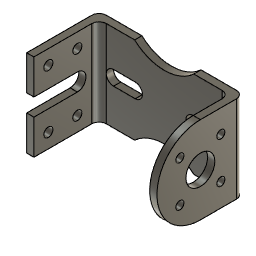
Tarea09_Ej2_jaalobuela (Autodesk Fusion 360 design; units mm, degrees)
Autodesk Fusion 360 part; units mm, degrees
sketch "Sketch1" plane through (0, 0, 0) normal (1, 0, 0) x (0, 1, 0)
  line L0 (-24.0301, 61.9141) -> (25.9699, 61.9141)
  line L1 (25.9699, 61.9141) -> (25.9699, 1.9141)
  line L2 (25.9699, 1.9141) -> (-24.0301, 1.9141)
  line L3 (-24.0301, 1.9141) -> (-29, 1.9141) construction
  line L4 (5.9699, 37.9141) -> (-24.0301, 37.9141)
  line L5 (5.9699, 25.9141) -> (-24.0301, 25.9141)
  arc A0 (5.9699, 25.9141) -> (5.9699, 37.9141) centre (5.9699, 31.9141) ccw
  line L6 (-24.0301, 1.9141) -> (-24.0301, 25.9141)
  line L7 (-24.0301, 37.9141) -> (-24.0301, 61.9141)
  line L8 (-24.0301, 61.9141) -> (-28, 61.9141) construction
  circle A1 centre (5.9699, 51.9141) radius 3.15
  circle A2 centre (-14.0301, 51.9141) radius 3.15
  circle A3 centre (5.9699, 11.9141) radius 3.15
  circle A4 centre (-14.0301, 11.9141) radius 3.15
  dimension "d1" = 50
  dimension "d2" = 60
  constraint horizontal L0
  constraint vertical L1
  constraint horizontal L2
  constraint vertical L6
  constraint perpendicular L3 L6
  constraint tangent L4 A0
  constraint perpendicular L4 L6
  constraint tangent L5 A0
  constraint perpendicular L5 L6
  constraint coincident L4.end L6
  constraint collinear L6 L7
  constraint perpendicular L7 L8
  measures "d1" distance of L0.start L0.end
  measures "d2" distance of L0.start L2.end
extrude "Extrude1" add sketch "Sketch1" along normal blind 5 makes body 1
sketch "Sketch2" plane through (0, 0, 0) normal (0, 1, 0) x (1, 0, 0)
  line L0 (148.3482, -63.5983) -> (148.3482, -3.5983)
  line L1 (48.3482, -3.5983) -> (48.3482, -63.5983)
  line L2 (148.3482, -63.5983) -> (148.3482, -72.5822) construction
  arc A0 (118.7443, -63.5983) -> (77.9522, -63.5983) centre (98.3482, -85.5983) ccw
  line L3 (48.3482, -63.5983) -> (77.9522, -63.5983)
  line L4 (118.7443, -63.5983) -> (148.3482, -63.5983)
  arc A1 (77.9522, -3.5983) -> (118.7443, -3.5983) centre (98.3482, 18.4017) ccw
  line L5 (148.3482, -3.5983) -> (118.7443, -3.5983)
  line L6 (77.9522, -3.5983) -> (48.3482, -3.5983)
  line L7 (63.3482, -38.5983) -> (78.3482, -38.5983)
  line L8 (78.3482, -28.5983) -> (63.3482, -28.5983)
  arc A2 (63.3482, -28.5983) -> (63.3482, -38.5983) centre (63.3482, -33.5983) ccw
  arc A3 (78.3482, -38.5983) -> (78.3482, -28.5983) centre (78.3482, -33.5983) ccw
  arc A4 (118.3482, -28.5983) -> (118.3482, -38.5983) centre (118.3482, -33.5983) ccw
  line L9 (118.3482, -28.5983) -> (133.3482, -28.5983)
  line L10 (133.3482, -38.5983) -> (118.3482, -38.5983)
  arc A5 (133.3482, -38.5983) -> (133.3482, -28.5983) centre (133.3482, -33.5983) ccw
  dimension "d12" = 100
  dimension "d13" = 60
  constraint horizontal L3
  constraint vertical L0
  constraint horizontal L5
  constraint vertical L1
  constraint perpendicular L2 L3
  constraint coincident A0.start L3
  constraint collinear L3 L4
  constraint collinear L5 L6
  constraint tangent L7 A3
  constraint tangent L8 A2
  measures "d12" distance of L1.end L0.start
  measures "d13" distance of L1.end L1.start
extrude "Extrude2" add sketch "Sketch2" along normal blind 5 separate body makes body 2
move_body "Move1" bodies 2 to x (1, 0, 0) y (0, 1, 0) z (0, 0, 1) at (-43.3482, 20.9699, -1.6842)
move_body "Move2" bodies 2 to x (1, 0, 0) y (0, 1, 0) z (0, 0, 1) at (-5, 0, 0)
sketch "Sketch3" plane through (0, 20.9699, 0) normal (0, -1, 0) x (1, 0, 0)
  arc A0 (30, 26.9141) -> (30, 36.9141) centre (30, 31.9141) ccw
  line L0 (30, 26.9141) -> (15, 26.9141)
  arc A1 (15, 36.9141) -> (15, 26.9141) centre (15, 31.9141) ccw
  line L1 (15, 36.9141) -> (30, 36.9141)
  arc A2 (70, 36.9141) -> (70, 26.9141) centre (70, 31.9141) ccw
  line L2 (70, 36.9141) -> (85, 36.9141)
  arc A3 (85, 26.9141) -> (85, 36.9141) centre (85, 31.9141) ccw
  line L3 (85, 26.9141) -> (70, 26.9141)
  line L4 (100, 61.9141) -> (70.3961, 61.9141)
  arc A4 (29.6039, 61.9141) -> (70.3961, 61.9141) centre (50, 83.9141) ccw
  line L5 (29.6039, 61.9141) -> (0, 61.9141)
  line L6 (0, 61.9141) -> (0, 1.9141)
  line L7 (0, 1.9141) -> (29.6039, 1.9141)
  arc A5 (70.3961, 1.9141) -> (29.6039, 1.9141) centre (50, -20.0859) ccw
  line L8 (70.3961, 1.9141) -> (100, 1.9141)
  line L9 (100, 1.9141) -> (100, 61.9141)
sketch "Sketch4" plane through (0, 0, 0) normal (1, 0, 0) x (0, 1, 0)
  line L0 (125, 0) -> (95, 0)
  line L1 (95, 60) -> (125, 60)
  line L2 (125, 60) -> (125, 0)
  circle A0 centre (95, 30) radius 10
  line L3 (200, 45) -> (200, 15) construction
  line L4 (200, 30) -> (215, 30) construction
  line L5 (200, 30) -> (185, 30) construction
  line L6 (200, 50) -> (220, 50) construction
  line L7 (200, 50) -> (180, 50) construction
  line L8 (200, 10) -> (220, 10) construction
  line L9 (200, 10) -> (180, 10) construction
  circle A1 centre (220, 50) radius 2.8 construction
  circle A2 centre (180, 50) radius 2.8 construction
  circle A3 centre (220, 10) radius 2.8 construction
  circle A4 centre (180, 10) radius 2.8 construction
  arc A5 (95, 60) -> (95, 0) centre (95, 30) ccw
  line L10 (200, 45) -> (215, 45) construction
  line L11 (200, 45) -> (185, 45) construction
  line L12 (200, 15) -> (215, 15) construction
  line L13 (200, 15) -> (185, 15) construction
  circle A6 centre (185, 45) radius 2.8 construction
  circle A7 centre (215, 45) radius 2.8 construction
  circle A8 centre (185, 15) radius 2.8 construction
  circle A9 centre (215, 15) radius 2.8 construction
  circle A10 centre (109.1421, 44.1421) radius 2.8
  circle A11 centre (80.8579, 44.1421) radius 2.8
  circle A12 centre (80.8579, 15.8579) radius 2.8
  circle A13 centre (109.1421, 15.8579) radius 2.8
  line L14 (95, 30) -> (115, 30) construction
  dimension "d27" = 60
  dimension "d37" = 5.6
  dimension "d38" = 5.6
  dimension "d39" = 30
  dimension "d40" = 15
  dimension "d41" = 15
  dimension "d42" = 15
  dimension "d43" = 15
  dimension "d44" = 15
  dimension "d45" = 15
  dimension "d46" = 5.6
  dimension "d47" = 5.6
  dimension "d48" = 5.6
  dimension "d49" = 5.6
  dimension "d50" = 5.6
  dimension "d51" = 5.6
  dimension "d52" = 5.6
  dimension "d53" = 5.6
  constraint horizontal L0
  constraint horizontal L1
  constraint vertical L2
  constraint concentric A0 A5
  constraint vertical L3
  constraint midpoint L3 L4.start
  constraint perpendicular L3 L4
  constraint perpendicular L3 L5
  constraint coincident L6.end A1.centre
  constraint coincident L7.end A2.centre
  constraint symmetric L4 A1 A3
  constraint symmetric L4 A2 A4
  constraint coincident L11.end A6.centre
  constraint coincident L10.end A7.centre
  constraint coincident L13.end A8.centre
  constraint coincident L12.end A9.centre
  constraint horizontal L14
  constraint coincident A0.centre A5.centre
  measures "d27" distance of L0.start L1.end
  measures "d37" diameter of A1
  measures "d38" diameter of A2
  measures "d39" distance of L3.start L3.end
  measures "d40" distance of L4.start L4.end
  measures "d41" distance of L4.start L5.end
  measures "d42" distance of L10.end L3.start
  measures "d43" distance of L3.start L11.end
  measures "d44" distance of L3.end L12.end
  measures "d45" distance of L3.end L13.end
  measures "d46" diameter of A6
  measures "d47" diameter of A7
  measures "d48" diameter of A8
  measures "d49" diameter of A9
  measures "d50" diameter of A11
  measures "d51" diameter of A10
  measures "d52" diameter of A12
  measures "d53" diameter of A13
extrude "Extrude3" add sketch "Sketch4" along normal blind 5 separate body makes body 3
move_body "Move3" bodies 3 to x (1, 0, 0) y (0, 1, 0) z (0, 0, 1) at (100, -104.0301, 1.9141)
move_body "Move4" bodies 3 to x (1, 0, 0) y (0, 1, 0) z (0, 0, 1) at (-5, 5, 0)
copy_body "CopyPasteBodies1" bodies 2 1 3 makes body 4 makes body 5 makes body 6
move_body "Move5" bodies 4 5 6 to x (1, 0, 0) y (0, 1, 0) z (0, 0, 1) at (220, 0, 0)
combine "Combine1" operation add target body 5 tool bodies 6 4
fillet "Fillet1" radius 5 4 edges at (225, 20.9699, 31.9141) (315, 20.9699, 31.9141) (220, 25.9699, 31.9141) (320, 25.9699, 31.9141) on bodies 5
hidden bodies 1 2 3
